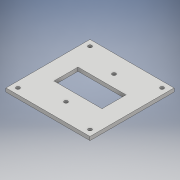
# Autodesk Inventor part: Servo Holder TOP
Saved by Autodesk Inventor 2017 (Build 210142000, 142)
## iProperties
Created: 2021-03-08
Part Number: Servo Holder TOP
Material: Generic
Document SubType Name: Modeling
Designer: Lenovo Y900
Density: 1 g/cm^3
Appearance: Default
Author: Lenovo Y900
Autodesk Inventor part; units mm, degrees
ref_plane "YZ Plane" through (0, 0, 0) normal (1, 0, 0) x (0, 1, 0)
ref_plane "XZ Plane" through (0, 0, 0) normal (0, 1, 0) x (-1, 0, 0)
ref_plane "XY Plane" through (0, 0, 0) normal (0, 0, 1) x (1, 0, 0)
sketch "Sketch1" plane through (0, 0, 0) normal (0, 0, 1) x (1, 0, 0)
  line L0 (-20, 10) -> (20, 10)
  line L1 (20, 10) -> (20, -10)
  line L2 (20, -10) -> (-20, -10)
  line L3 (-20, -10) -> (-20, 10)
  line L4 (-20, 10) -> (20, -10) construction
  line L5 (20, 10) -> (-20, -10) construction
  line L6 (20, 0) -> (30, 0)
  line L7 (35, -35) -> (-35, -35)
  line L8 (-35, -35) -> (-35, 35)
  line L9 (-35, 35) -> (35, 35)
  line L10 (35, 35) -> (35, -35)
  line L11 (35, -35) -> (-35, 35) construction
  line L12 (-35, -35) -> (35, 35) construction
  line L13 (30, -30) -> (-30, 30) construction
  line L14 (-30, -30) -> (30, 30) construction
  circle A0 centre (-30, 30) radius 1.5
  circle A1 centre (30, 30) radius 1.5
  circle A2 centre (-30, -30) radius 1.5
  circle A3 centre (30, -30) radius 1.5
  line L15 (0, 10) -> (0, 20)
  line L16 (0, -10) -> (0, -20)
  circle A4 centre (0, 20) radius 1.5
  circle A5 centre (0, -20) radius 1.5
  point P0 (0, 0)
  dimension "d0" = 40
  dimension "d1" = 20
  dimension "d2" = 10
  dimension "d3" = 70
  dimension "d4" = 70
  dimension "d9" = 3
  dimension "d10" = 3
  dimension "d11" = 3
  dimension "d12" = 3
  dimension "d15" = 10
  dimension "d16" = 10
  dimension "d17" = 3
  dimension "d18" = 3
  constraints: 34 end point, 9 midpoint, 6 centre point, 6 coincident, 4 parallel, 3 horizontal, 2 perpendicular, 2 vertical, 1 point on line
  measures "d0" distance of L1.end L2.end
  measures "d1" distance of L0.end L1.end
  measures "d2" distance of L6.start L6.end
  measures "d3" distance of L8.end L9.end
  measures "d4" distance of L7.end L8.end
  measures "d9" diameter of A0
  measures "d10" diameter of A1
  measures "d11" diameter of A2
  measures "d12" diameter of A3
  measures "d15" distance of L15.start L15.end
  measures "d16" distance of L16.start L16.end
  measures "d17" diameter of A4
  measures "d18" diameter of A5
extrude "Extrusion3" add sketch "Sketch1" along normal blind 3
body "Solid3"
